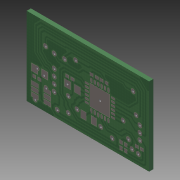
# Autodesk Inventor part: Audio_module_PCB
Saved by Autodesk Inventor 2013 (Build 170138000, 138)
## iProperties
Created: 2015-07-03
Part Number: Audio_module_PCB
Material: Ogólny
Document SubType Name: Modeling
Designer: terg
Density: 1 g/cm^3
Author: terg
Autodesk Inventor part; units mm, degrees
ref_plane "YZ Plane" through (0, 0, 0) normal (1, 0, 0) x (0, 1, 0)
ref_plane "XZ Plane" through (0, 0, 0) normal (0, 1, 0) x (-1, 0, 0)
ref_plane "XY Plane" through (0, 0, 0) normal (0, 0, 1) x (1, 0, 0)
sketch "Szkic1" plane through (0, 0, 0) normal (0, 1, 0) x (-1, 0, 0)
  line L0 (0, 0) -> (-23.5, 0)
  line L1 (-23.5, 0) -> (-23.5, -15)
  line L2 (-23.5, -15) -> (0, -15)
  line L3 (0, -15) -> (0, 0)
  dimension "d0" = 23.5
  dimension "d1" = 15
  constraints: 8 end point, 2 parallel, 1 horizontal, 1 perpendicular
  measures "d0" distance of L2.end L1.end
  measures "d1" distance of L1.end L0.end
extrude "Wyciągnięcie proste1" add sketch "Szkic1" along normal blind 0.8
sketch "Szkic2" plane through (0, 0.8, 0) normal (0, 1, 0) x (1, 0, 0)
  line L0 (0, 0) -> (23.5, 0) projected
  line L1 (23.5, 0) -> (23.5, 15) projected
  line L2 (23.5, 15) -> (0, 15) projected
  line L3 (0, 15) -> (0, 0) projected
  line L4 (-0.025, 15) -> (23.525, 15) construction
  line L5 (23.525, 15) -> (23.525, 0) construction
  line L6 (23.525, 0) -> (-0.025, 0) construction
  line L7 (-0.025, 0) -> (-0.025, 15) construction
  dimension "d9" = 0
  dimension "d10" = -0.025
  dimension "d11" = 0
  dimension "d12" = -0.025
  constraints: 2 other
  measures "d9" distance between parallel lines of L2 L4
  measures "d10" distance between parallel lines of L1 L5
  measures "d11" distance between parallel lines of L0 L6
  measures "d12" distance between parallel lines of L3 L7
decal "Pokrycie bitmapą1"
sketch "Szkic3" plane through (0, 0, 0) normal (0, -1, 0) x (1, 0, 0)
  line L0 (0, 0) -> (23.5, 0) projected
  line L1 (0, -15) -> (0, 0) projected
  line L2 (23.5, -15) -> (0, -15) projected
  line L3 (23.5, 0) -> (23.5, -15) projected
  line L4 (23.5185, -15) -> (-0.0185, -15) construction
  line L5 (-0.0185, -15) -> (-0.0185, 0) construction
  line L6 (-0.0185, 0) -> (23.5185, 0) construction
  line L7 (23.5185, 0) -> (23.5185, -15) construction
  dimension "d34" = 0
  dimension "d35" = -0.0185
  dimension "d36" = 0
  dimension "d37" = -0.0185
  constraints: 2 other
  measures "d34" distance between parallel lines of L0 L6
  measures "d35" distance between parallel lines of L3 L7
  measures "d36" distance between parallel lines of L2 L4
  measures "d37" distance between parallel lines of L1 L5
decal "Pokrycie bitmapą2"
sketch "Szkic4" plane through (0, 0.8, 0) normal (0, 1, 0) x (1, 0, 0)
  point P0 (1.6054, 13.9495)
  point P1 (3.7304, 11.0125)
  point P2 (5.2862, 10.8455)
  point P3 (5.2862, 9.5781)
  point P4 (3.2902, 9.0924)
  point P5 (5.2862, 8.2728)
  point P6 (5.2862, 6.9902)
  point P7 (7.7906, 8.2728)
  point P8 (7.9804, 10.2308)
  point P9 (2.0001, 8.5612)
  point P10 (5.2862, 4.4858)
  point P11 (3.6166, 4.0912)
  point P12 (7.2746, 4.4403)
  point P13 (9.3996, 3.5447)
  point P14 (14.0657, 7.9031)
  point P15 (14.1988, 12.2076)
  point P16 (16.3962, 13.0194)
  point P17 (19.5083, 11.6176)
  point P18 (20.1957, 12.9274)
  point P19 (21.4031, 13.1271)
  point P20 (21.6981, 10.7093)
  point P21 (21.6981, 9.4618)
  point P22 (18.4921, 8.9927)
  point P23 (21.6981, 8.19)
  point P24 (20.9824, 6.8796)
  point P25 (20.3947, 3.1866)
  point P26 (5.8639, 13.5455)
  point P27 (7.9804, 13.0194)
  point P28 (9.6589, 11.5547)
hole "Otwór1" at (1.6054, 0.8, -13.9495) at (3.7304, 0.8, -11.0125) at (5.2862, 0.8, -10.8455) at (5.2862, 0.8, -9.5781) at (3.2902, 0.8, -9.0924) at (5.2862, 0.8, -8.2728) at (5.2862, 0.8, -6.9902) at (7.7906, 0.8, -8.2728) at (7.9804, 0.8, -10.2308) at (2.0001, 0.8, -8.5612) at (5.2862, 0.8, -4.4858) at (3.6166, 0.8, -4.0912) at (7.2746, 0.8, -4.4403) at (9.3996, 0.8, -3.5447) at (14.0657, 0.8, -7.9031) at (14.1988, 0.8, -12.2076) at (16.3962, 0.8, -13.0194) at (19.5083, 0.8, -11.6176) at (20.1957, 0.8, -12.9274) at (21.4031, 0.8, -13.1271) at (21.6981, 0.8, -10.7093) at (21.6981, 0.8, -9.4618) at (18.4921, 0.8, -8.9927) at (21.6981, 0.8, -8.19) at (20.9824, 0.8, -6.8796) at (20.3947, 0.8, -3.1866) at (5.8639, 0.8, -13.5455) at (7.9804, 0.8, -13.0194) at (9.6589, 0.8, -11.5547) direction (0, -1, 0) diameter 0.4 depth 8
equation "\"d10\" = d12"
equation "\"d35\" = d37"
